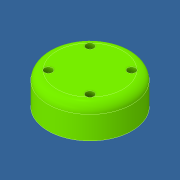
# Autodesk Inventor part: MotorCoverN24_3
Saved by Autodesk Inventor 2016 (Build 200138000, 138)
## iProperties
Created: 2015-09-10
Part Number: MotorCoverN24_3
Material: ABS-Kunststoff
Document SubType Name: Modeling
Designer: 4ndreas
Density: 1.06 g/cm^3
Appearance: Glatt - grün
Mass: 123.659 g
Surface Area: 337.654 cm^2
Volume: 116.659 cm^3
Author: 4ndreas
Autodesk Inventor part; units mm, degrees
ref_plane "YZ Plane" through (0, 0, 0) normal (1, 0, 0) x (0, 1, 0)
ref_plane "XZ Plane" through (0, 0, 0) normal (0, 1, 0) x (-1, 0, 0)
sketch "Skizze1" plane through (0, 0, 0) normal (0, 0, 1) x (1, 0, 0)
  line L0 (24.616, 19.6663) -> (20.7123, 20.7123) projected
  line L1 (20.7123, 20.7123) -> (19.6663, 24.616) projected
  line L2 (19.6663, 24.616) -> (22.524, 27.4737) projected
  line L3 (22.524, 27.4737) -> (26.4277, 26.4277) projected
  line L4 (26.4277, 26.4277) -> (27.4737, 22.524) projected
  line L5 (27.4737, 22.524) -> (24.616, 19.6663) projected
  line L6 (-24.616, -19.6663) -> (-20.7123, -20.7123) projected
  line L7 (-20.7123, -20.7123) -> (-19.6663, -24.616) projected
  line L8 (-19.6663, -24.616) -> (-22.524, -27.4737) projected
  line L9 (-22.524, -27.4737) -> (-26.4277, -26.4277) projected
  line L10 (-26.4277, -26.4277) -> (-27.4737, -22.524) projected
  line L11 (-27.4737, -22.524) -> (-24.616, -19.6663) projected
  line L12 (-20.7123, 20.7123) -> (-24.616, 19.6663) projected
  line L13 (-24.616, 19.6663) -> (-27.4737, 22.524) projected
  line L14 (-27.4737, 22.524) -> (-26.4277, 26.4277) projected
  line L15 (-26.4277, 26.4277) -> (-22.524, 27.4737) projected
  line L16 (-22.524, 27.4737) -> (-19.6663, 24.616) projected
  line L17 (-19.6663, 24.616) -> (-20.7123, 20.7123) projected
  line L18 (19.6663, -24.616) -> (20.7123, -20.7123) projected
  line L19 (20.7123, -20.7123) -> (24.616, -19.6663) projected
  line L20 (24.616, -19.6663) -> (27.4737, -22.524) projected
  line L21 (27.4737, -22.524) -> (26.4277, -26.4277) projected
  line L22 (26.4277, -26.4277) -> (22.524, -27.4737) projected
  line L23 (22.524, -27.4737) -> (19.6663, -24.616) projected
  arc A0 (-23.57, 19.32) -> (-19.32, 23.57) centre (-23.57, 23.57) ccw projected
  line L24 (-19.32, 23.57) -> (-19.32, 32.18) projected
  line L25 (-19.32, 32.18) -> (19.32, 32.18) projected
  line L26 (19.32, 32.18) -> (19.32, 23.57) projected
  arc A1 (19.32, 23.57) -> (23.57, 19.32) centre (23.57, 23.57) ccw projected
  line L27 (23.57, 19.32) -> (32.18, 19.32) projected
  line L28 (32.18, 19.32) -> (32.18, -19.32) projected
  line L29 (32.18, -19.32) -> (23.57, -19.32) projected
  arc A2 (23.57, -19.32) -> (19.32, -23.57) centre (23.57, -23.57) ccw projected
  line L30 (19.32, -23.57) -> (19.32, -32.18) projected
  line L31 (19.32, -32.18) -> (-19.32, -32.18) projected
  line L32 (-19.32, -32.18) -> (-19.32, -23.57) projected
  arc A3 (-19.32, -23.57) -> (-23.57, -19.32) centre (-23.57, -23.57) ccw projected
  line L33 (-23.57, -19.32) -> (-32.18, -19.32) projected
  line L34 (-32.18, -19.32) -> (-32.18, 19.32) projected
  line L35 (-32.18, 19.32) -> (-23.57, 19.32) projected
  circle A4 centre (0, 0) radius 47.5
  circle A5 centre (23.57, -23.57) radius 2
  circle A6 centre (23.57, 23.57) radius 2
  circle A7 centre (-23.57, 23.57) radius 2
  circle A8 centre (-23.57, -23.57) radius 2
  arc A9 (32.18, -19.32) -> (32.18, 19.32) centre (0, 0) ccw
  arc A10 (-19.32, -32.18) -> (19.32, -32.18) centre (0, 0) ccw
  arc A11 (-32.18, 19.32) -> (-32.18, -19.32) centre (0, 0) ccw
  arc A12 (19.32, 32.18) -> (-19.32, 32.18) centre (0, 0) ccw
  point P0 (0, 0)
  dimension "d0" = 4
  dimension "d40" = 95
  constraints: 9 centre point, 8 coincident, 8 point on circle, 3 equal radius
  measures "d0" diameter of A5
  measures "d40" diameter of A4
extrude "Extrusion1" add sketch "Skizze1" along normal blind 32 contours L0 L1 L2 L3 L4 L5 | L6 L7 L8 L9 L10 L11 | L12 L13 L14 L15 L16 L17 | L18 L19 L20 L21 L22 L23 | A4
ref_plane "Arbeitsebene1" through (0, 0, 0) normal (1, 0, 0) x (0, 0, 1)
sketch "Skizze9" plane through (0, 0, 32) normal (0, 0, 1) x (1, 0, 0)
  circle A0 centre (23.57, -23.57) radius 2 projected
  circle A1 centre (-23.57, 23.57) radius 2 projected
  circle A2 centre (-23.57, -23.57) radius 2 projected
  circle A3 centre (23.57, 23.57) radius 2 projected
  circle A4 centre (0, 0) radius 47.5 projected
  line L0 (32.18, -19.32) -> (23.57, -19.32) projected
  arc A5 (23.57, -19.32) -> (19.32, -23.57) centre (23.57, -23.57) ccw projected
  line L1 (19.32, -23.57) -> (19.32, -32.18) projected
  arc A6 (-19.32, -32.18) -> (19.32, -32.18) centre (0, 0) ccw projected
  line L2 (-19.32, -32.18) -> (-19.32, -23.57) projected
  arc A7 (-19.32, -23.57) -> (-23.57, -19.32) centre (-23.57, -23.57) ccw projected
  line L3 (-23.57, -19.32) -> (-32.18, -19.32) projected
  arc A8 (-32.18, 19.32) -> (-32.18, -19.32) centre (0, 0) ccw projected
  line L4 (-32.18, 19.32) -> (-23.57, 19.32) projected
  arc A9 (-23.57, 19.32) -> (-19.32, 23.57) centre (-23.57, 23.57) ccw projected
  line L5 (-19.32, 23.57) -> (-19.32, 32.18) projected
  arc A10 (19.32, 32.18) -> (-19.32, 32.18) centre (0, 0) ccw projected
  line L6 (19.32, 32.18) -> (19.32, 23.57) projected
  arc A11 (19.32, 23.57) -> (23.57, 19.32) centre (23.57, 23.57) ccw projected
  line L7 (23.57, 19.32) -> (32.18, 19.32) projected
  arc A12 (32.18, -19.32) -> (32.18, 19.32) centre (0, 0) ccw projected
  point P0 (0, 0)
extrude "Extrusion6" add sketch "Skizze9" along normal blind 4 contours A4 | L0 A5 L1 A6 L2 A7 L3 A8 L4 A9 L5 A10 L6 A11 L7 A12
fillet "Rundung3" radius 10 1 edges at (-47.5, 0, 36)
sketch "Skizze10" plane through (0, 0, 0) normal (0, 0, -1) x (-1, 0, 0)
  circle A0 centre (-23.57, -23.57) radius 2 projected
  circle A1 centre (23.57, 23.57) radius 2 projected
  circle A2 centre (23.57, -23.57) radius 2 projected
  circle A3 centre (-23.57, 23.57) radius 2 projected
  line L0 (-23.57, -19.32) -> (-32.18, -19.32) projected
  arc A4 (-32.18, 19.32) -> (-32.18, -19.32) centre (0, 0) ccw projected
  line L1 (-32.18, 19.32) -> (-23.57, 19.32) projected
  arc A5 (-23.57, 19.32) -> (-19.32, 23.57) centre (-23.57, 23.57) ccw projected
  line L2 (-19.32, 23.57) -> (-19.32, 32.18) projected
  arc A6 (19.32, 32.18) -> (-19.32, 32.18) centre (0, 0) ccw projected
  line L3 (19.32, 32.18) -> (19.32, 23.57) projected
  arc A7 (19.32, 23.57) -> (23.57, 19.32) centre (23.57, 23.57) ccw projected
  line L4 (23.57, 19.32) -> (32.18, 19.32) projected
  arc A8 (32.18, -19.32) -> (32.18, 19.32) centre (0, 0) ccw projected
  line L5 (32.18, -19.32) -> (23.57, -19.32) projected
  arc A9 (23.57, -19.32) -> (19.32, -23.57) centre (23.57, -23.57) ccw projected
  line L6 (19.32, -23.57) -> (19.32, -32.18) projected
  arc A10 (-19.32, -32.18) -> (19.32, -32.18) centre (0, 0) ccw projected
  line L7 (-19.32, -32.18) -> (-19.32, -23.57) projected
  arc A11 (-19.32, -23.57) -> (-23.57, -19.32) centre (-23.57, -23.57) ccw projected
  circle A12 centre (0, 0) radius 47.5 projected
  point P0 (0, 0)
fillet "Rundung4" radius 5 12 edges at (20.5648, 20.5648, 32) (27.875, 19.32, 32) (19.32, 27.875, 32) (19.32, -27.875, 32) (27.875, -19.32, 32) (20.5648, -20.5648, 32) (-27.875, -19.32, 32) (-19.32, -27.875, 32) (-20.5648, -20.5648, 32) (-19.32, 27.875, 32) (-27.875, 19.32, 32) (-20.5648, 20.5648, 32)
sketch "Skizze11" plane through (0, 0, 36) normal (0, 0, 1) x (1, 0, 0)
  circle A0 centre (23.57, -23.57) radius 2 projected
  circle A1 centre (-23.57, 23.57) radius 2 projected
  circle A2 centre (-23.57, -23.57) radius 2 projected
  circle A3 centre (23.57, 23.57) radius 2 projected
  circle A4 centre (0, 0) radius 37.5 projected
  point P0 (0, 0)
hole "Bohrung2" at (-23.57, 23.57, 36) at (23.57, 23.57, 36) at (23.57, -23.57, 36) at (-23.57, -23.57, 36) direction (0, 0, -1) diameter 4.2 end through all counterbore diameter 9 counterbore depth 6
